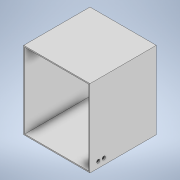
# Autodesk Inventor part: mouse_SP_inner
Saved by Autodesk Inventor 2020 (Build 240168000, 168)
## iProperties
Created: 2019-06-13
Part Number: mouse_SP_inner
Material: Generic
Document SubType Name: Modeling
Designer: Dammy
Density: 1 g/cm^3
Appearance: Default
Author: Dammy
Autodesk Inventor part; units mm, degrees
ref_plane "YZ Plane" through (0, 0, 0) normal (1, 0, 0) x (0, 1, 0)
ref_plane "XZ Plane" through (0, 0, 0) normal (0, 1, 0) x (-1, 0, 0)
ref_plane "XY Plane" through (0, 0, 0) normal (0, 0, 1) x (1, 0, 0)
sketch "Sketch2" plane through (0, 0, 0) normal (0, 0, 1) x (1, 0, 0)
  line L0 (150, -175) -> (-150, -175)
  line L1 (-150, -175) -> (-150, 175)
  line L2 (-150, 175) -> (150, 175)
  line L3 (150, 175) -> (150, -175)
  line L4 (150, -175) -> (-150, 175) construction
  line L5 (-150, -175) -> (150, 175) construction
  point P0 (0, 0)
  dimension "d0" = 300
  dimension "d1" = 350
  constraints: 12 end point, 2 midpoint, 2 parallel, 1 horizontal, 1 perpendicular
  measures "d0" distance of L1.end L2.end
  measures "d1" distance of L0.end L1.end
extrude "Base" add sketch "Sketch2" along normal blind 300
shell "Shell1" thickness 5 removed faces 1 at (50, -58.3333, 300)
sketch "Sketch3" plane through (150, -175, 0) normal (1, 0, 0) x (0, 0, -1)
  circle A0 centre (-262.5, 27.5) radius 7.5
  line L0 (-300, 350) -> (-300, 0) projected
  line L1 (0, 0) -> (-300, 0) projected
  circle A1 centre (-237.5, 27.5) radius 7.5
  point P0 (0, 175)
  dimension "d5" = 15
  dimension "d9" = 37.5
  dimension "d10" = 27.5
  dimension "d13" = 25
  constraints: 2 centre point, 1 horizontal, 2 other
  measures "d5" diameter of A0
  measures "d9" distance from line of L0 A0.centre
  measures "d10" distance from line of L1 A0.centre
  measures "d13" distance of A0.centre A1.centre
extrude "Wire holes" cut sketch "Sketch3" against normal up to surface (5 mm away)
sketch "Sketch4" plane through (0, 0, 0) normal (0, 0, -1) x (-1, 0, 0)
  circle A0 centre (-96.967, -121.967) radius 25
  line L0 (-150, -175) -> (-96.967, -121.967) construction
  line L1 (-150, -175) -> (-75, -175) construction
  point P0 (0, 0)
  dimension "d20" = 50
  dimension "d21" = 75
  dimension "d22" = 45
  constraints: 4 end point, 1 centre point, 1 coincident, 1 equal length, 1 horizontal
  measures "d20" diameter of A0
  measures "d21" distance of L0.start L0.end
  measures "d22" angle of L1 L0
extrude "Exhaust" cut sketch "Sketch4" against normal up to surface (5 mm away)
body "Solid1"
